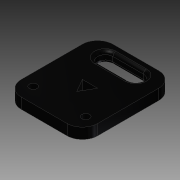
# Autodesk Inventor part: tubing_alignment_arm
Saved by Autodesk Inventor 2015 (Build 190159000, 159)
## iProperties
Created: 2017-04-04
Part Number: tubing_alignment_arm
Material: Acetal Resin, Black
Document SubType Name: Modeling
Designer: Guy
Density: 1.425 g/cm^3
Appearance: Smooth - Black
Author: Guy
Autodesk Inventor part; units mm, degrees
ref_plane "YZ Plane" through (0, 0, 0) normal (1, 0, 0) x (0, 1, 0)
ref_plane "XZ Plane" through (0, 0, 0) normal (0, 1, 0) x (-1, 0, 0)
ref_plane "XY Plane" through (0, 0, 0) normal (0, 0, 1) x (1, 0, 0)
sketch "Sketch1" plane through (0, 0, 0) normal (0, 0, 1) x (1, 0, 0)
  line L0 (0, 0) -> (50, 0)
  line L1 (50, 0) -> (50, 60)
  line L2 (50, 60) -> (0, 60)
  line L3 (0, 60) -> (0, 0)
  dimension "d0" = 50
  dimension "d1" = 60
  constraints: 8 end point, 2 parallel, 1 horizontal, 1 perpendicular
  measures "d0" distance of L0.start L0.end
  measures "d1" distance of L2.end L0.start
extrude "Extrusion1" add sketch "Sketch1" along normal blind 7
sketch "Sketch2" plane through (0, 0, 7) normal (0, 0, 1) x (1, 0, 0)
  circle A0 centre (7.825, 10) radius 2.5
  circle A1 centre (42.175, 10) radius 2.5
  line L0 (0, 0) -> (50, 0) projected
  line L1 (50, 0) -> (50, 60) projected
  dimension "d4" = 5
  dimension "d5" = 5
  dimension "d6" = 34.35
  dimension "d9" = 10
  dimension "d10" = 10
  dimension "d11" = 50
  dimension "d12" = 7.825
  constraints: 2 centre point
  measures "d4" diameter of A1
  measures "d5" diameter of A0
  measures "d6" distance of A1.centre A0.centre
  measures "d9" distance from line of L0 A0.centre
  measures "d10" distance from line of L0 A1.centre
  measures "d11" distance of L0.start L0.end
  measures "d12" distance from line of A1.centre L1
extrude "Extrusion2" cut sketch "Sketch2" against normal up to next
sketch "Sketch3" plane through (0, 0, 7) normal (0, 0, 1) x (1, 0, 0)
  arc A0 (15, 55) -> (15, 45) centre (15, 50) ccw
  arc A1 (35, 45) -> (35, 55) centre (35, 50) ccw
  line L0 (15, 55) -> (35, 55)
  line L1 (15, 45) -> (35, 45)
  line L2 (50, 60) -> (0, 60) projected
  line L3 (50, 0) -> (50, 60) projected
  line L4 (0, 60) -> (0, 0) projected
  dimension "d15" = 10
  dimension "d16" = 10
  dimension "d19" = 20
  dimension "d20" = 50
  dimension "d21" = 15
  constraints: 4 end point, 4 point on circle, 4 tangent, 2 centre point, 2 parallel
  measures "d15" diameter of A1
  measures "d16" distance from line of A1.centre L2
  measures "d19" distance of A0.centre A1.centre
  measures "d20" distance of L2.start L2.end
  measures "d21" distance from line of A1.centre L3
extrude "Extrusion3" cut sketch "Sketch3" against normal up to next
fillet "Fillet1" radius 10 4 edges at (0, 60, 3.5) (50, 60, 3.5) (50, 0, 3.5) (0, 0, 3.5)
sketch "Sketch4" plane through (0, 0, 7) normal (0, 0, 1) x (1, 0, 0)
  line L0 (25, 21.3397) -> (30, 30)
  line L1 (30, 30) -> (20, 30)
  line L2 (20, 30) -> (25, 21.3397)
  line L3 (35, 45) -> (15, 45) projected
  line L4 (0, 50) -> (0, 10) projected
  line L5 (10, 0) -> (40, 0) projected
  point P0 (0, 0)
  dimension "d23" = 60
  dimension "d24" = 60
  dimension "d25" = 10
  dimension "d26" = 20
  dimension "d27" = 30
  constraints: 6 end point, 1 horizontal, 1 parallel
  measures "d23" angle of L2 L1
  measures "d24" angle of L1 L0
  measures "d25" distance of L0.end L1.end
  measures "d26" distance from line of L4 L1.end
  measures "d27" distance from line of L5 L1.end
extrude "Extrusion4" cut sketch "Sketch4" against normal up to next
fillet "Fillet2" radius 2 8 edges at (25, 55, 7) (40, 50, 7) (25, 45, 7) (10, 50, 7) (25, 55, 0) (10, 50, 0) (25, 45, 0) (40, 50, 0)
equation "\"d10\" = d9"
equation "\"d12\" = -0.5 * d6 + 0.5 * d11"
equation "\"d19\" = 2 * d15"
equation "\"d21\" = -0.5 * d19 + 0.5 * d20"
body "Solid1"
